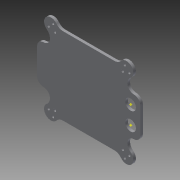
# Autodesk Inventor part: LowerPlatter
Saved by Autodesk Inventor 2015 (Build 190159000, 159)
## iProperties
Created: 2015-06-01
Part Number: LowerPlatter
Material: ABS Plastic
Document SubType Name: Modeling
Designer: Vu
Density: 1.06 g/cm^3
Appearance: Smooth - White
Mass: 73.1056 g
Surface Area: 379.193 cm^2
Volume: 68.9676 cm^3
Author: Vu
Autodesk Inventor part; units mm, degrees
ref_plane "YZ Plane" through (0, 0, 0) normal (1, 0, 0) x (0, 1, 0)
ref_plane "XZ Plane" through (0, 0, 0) normal (0, 1, 0) x (-1, 0, 0)
ref_plane "XY Plane" through (0, 0, 0) normal (0, 0, 1) x (1, 0, 0)
sketch "Sketch1" plane through (0, 0, 0) normal (0, 1, 0) x (-1, 0, 0)
  line L0 (-0.0023, 59.9989) -> (-40.0023, 59.9989)
  line L1 (-0.0023, 59.9989) -> (39.9977, 59.9989) construction
  line L2 (-60.0163, -0.0152) -> (-60.0163, 39.9848)
  line L3 (-60.0163, -0.0152) -> (-20.0163, -0.0152) construction
  line L4 (-60.0163, -0.0152) -> (-0.0023, -0.0152)
  line L5 (-0.0023, -0.0152) -> (-0.0023, 59.9989)
  arc A0 (-49.9687, 64.958) -> (-40.0023, 59.9989) centre (-40.0023, 72.4933) ccw
  arc A1 (-60.0163, 39.9848) -> (-64.9755, 49.9513) centre (-72.5108, 39.9848) ccw
  arc A2 (-49.9687, 64.958) -> (-64.9755, 49.9513) centre (-58.5144, 58.4969) ccw
  line L6 (-40.0023, 59.9989) -> (-40.0023, 59.4989)
  line L7 (-60.0163, 39.9848) -> (-59.5163, 39.9848)
  arc A3 (-59.5163, 39.9848) -> (-40.0023, 59.4989) centre (-59.5163, 59.4989) ccw
  line L8 (-60.0163, -0.0152) -> (-80.0163, -0.0152)
  line L9 (-80.0163, -0.0152) -> (-80.0163, 19.9848)
  arc A4 (-70, 30.0011) -> (-60.0163, 39.9848) centre (-70, 39.9848) ccw
  arc A5 (-70, 30.0011) -> (-80.0163, 19.9848) centre (-70, 19.9848) ccw
  line L10 (-60.0163, -40.0152) -> (-59.5163, -40.0152)
  arc A6 (-64.9755, -49.9816) -> (-60.0163, -40.0152) centre (-72.5108, -40.0152) ccw
  line L11 (-60.0163, -0.0152) -> (-60.0163, -40.0152)
  arc A7 (-64.9755, -49.9816) -> (-49.9687, -64.9884) centre (-58.5144, -58.5273) ccw
  arc A8 (-40.0023, -60.0292) -> (-49.9687, -64.9884) centre (-40.0023, -72.5237) ccw
  arc A9 (-40.0023, -59.5292) -> (-59.5163, -40.0152) centre (-59.5163, -59.5292) ccw
  line L12 (-40.0023, -60.0292) -> (-40.0023, -59.5292)
  line L13 (-0.0023, -60.0292) -> (-40.0023, -60.0292)
  line L14 (-0.0023, -0.0152) -> (-0.0023, -60.0292)
  arc A10 (-60.0163, -40.0152) -> (-70, -30.0315) centre (-70, -40.0152) ccw
  line L15 (-80.0163, -0.0152) -> (-80.0163, -20.0152)
  arc A11 (-80.0163, -20.0152) -> (-70, -30.0315) centre (-70, -20.0152) ccw
  arc A12 (80.0118, 19.9848) -> (69.9955, 30.0011) centre (69.9955, 19.9848) ccw
  line L16 (60.0118, -0.0152) -> (80.0118, -0.0152)
  line L17 (80.0118, -0.0152) -> (80.0118, 19.9848)
  line L18 (-0.0023, 59.9989) -> (-40.0023, 59.9989) construction
  line L19 (-0.0023, 59.9989) -> (39.9977, 59.9989)
  line L20 (60.0118, -0.0152) -> (60.0118, 39.9848)
  arc A13 (60.0118, 39.9848) -> (69.9955, 30.0011) centre (69.9955, 39.9848) ccw
  line L21 (60.0118, 39.9848) -> (59.5118, 39.9848)
  arc A14 (64.9709, 49.9513) -> (60.0118, 39.9848) centre (72.5063, 39.9848) ccw
  line L22 (60.0118, -0.0152) -> (20.0118, -0.0152) construction
  arc A15 (64.9709, 49.9513) -> (49.9642, 64.958) centre (58.5098, 58.4969) ccw
  arc A16 (39.9977, 59.4989) -> (59.5118, 39.9848) centre (59.5118, 59.4989) ccw
  line L23 (39.9977, 59.9989) -> (39.9977, 59.4989)
  arc A17 (39.9977, 59.9989) -> (49.9642, 64.958) centre (39.9977, 72.4933) ccw
  line L24 (60.0118, -0.0152) -> (-0.0023, -0.0152)
  line L25 (80.0118, -0.0152) -> (80.0118, -20.0152)
  arc A18 (69.9955, -30.0315) -> (80.0118, -20.0152) centre (69.9955, -20.0152) ccw
  arc A19 (69.9955, -30.0315) -> (60.0118, -40.0152) centre (69.9955, -40.0152) ccw
  line L26 (60.0118, -40.0152) -> (59.5118, -40.0152)
  line L27 (60.0118, -0.0152) -> (60.0118, -40.0152)
  arc A20 (60.0118, -40.0152) -> (64.9709, -49.9816) centre (72.5063, -40.0152) ccw
  arc A21 (59.5118, -40.0152) -> (39.9977, -59.5292) centre (59.5118, -59.5292) ccw
  arc A22 (49.9642, -64.9884) -> (64.9709, -49.9816) centre (58.5098, -58.5273) ccw
  line L28 (39.9977, -60.0292) -> (39.9977, -59.5292)
  arc A23 (49.9642, -64.9884) -> (39.9977, -60.0292) centre (39.9977, -72.5237) ccw
  line L29 (-0.0023, -60.0292) -> (39.9977, -60.0292)
  point P0 (0, 0)
  point P1 (-55.5, 62.5)
  point P2 (-62.5, 55.5)
  point P3 (-52.5, 52.5)
  point P4 (-52.5, -52.5303)
  point P5 (-62.5, -55.5303)
  point P6 (-55.5, -62.5303)
  point P7 (55.4955, -62.5303)
  point P8 (62.4955, -55.5303)
  point P9 (52.4955, -52.5303)
  point P10 (52.4955, 52.5)
  point P11 (62.4955, 55.5)
  point P12 (55.4955, 62.5)
  point P13 (-65, 13.9848)
  point P14 (-65, -14.0152)
  dimension "d0" = 40
  dimension "d1" = 180
  dimension "d2" = 40
  dimension "d3" = 90
  dimension "d4" = 12.4944
  dimension "d5" = 12.4944
  dimension "d6" = 0.5
  dimension "d7" = 0.5
  dimension "d8" = 20
  dimension "d9" = 20
  dimension "d42" = 14
  dimension "d43" = 14
  constraints: 60 end point, 56 symmetric about line, 48 point on circle, 24 centre point, 9 tangent, 6 horizontal, 2 equal length, 2 perpendicular, 2 vertical, 18 other
  measures "d0" distance of L0.start L0.end
  measures "d1" angle of L0 L1
  measures "d2" distance of L3.start L2.end
  measures "d3" angle of L3 L2
  measures "d4" radius of A0
  measures "d5" radius of A1
  measures "d6" distance of L0.end L6.end
  measures "d7" distance of L2.end L7.end
  measures "d8" distance of L3.start L8.end
  measures "d9" distance of L8.end L9.end
  measures "d42" distance from line of L8 point (-65, 13.985)
  measures "d43" distance from line of point (-65, -14.015) L8
extrude "Extrusion1" add sketch "Sketch1" along normal blind 4 contours L5 L4 L2 L7 A3 L6 L0 | L19 L23 A16 L21 L20 L24 L5 | L14 L13 L12 A9 L10 L11 L4 | L24 L27 L26 A21 L28 L29 L14 | L8 L9 A5 A4 L2 | L11 A10 A11 L15 L8 | L20 A13 A12 L17 L16 | L16 L25 A18 A19 L27
extrude "Extrusion2" add sketch "Sketch1" along normal blind 4 contours L6 A3 L7 A1 A2 A0 | A17 A15 A14 L21 A16 L23 | L10 A9 L12 A8 A7 A6 | L28 A21 L26 A20 A22 A23
hole "Hole1" at (65, 0, -14.0152) direction (0, 1, 0) diameter 16.5 end through all
hole "Hole2" at (65, 0, 13.9848) direction (0, 1, 0) diameter 16.5 end through all
hole "Hole3" at (-55.4955, 0, 62.5) at (-62.4955, 0, 55.5) at (-52.4955, 0, 52.5) at (-52.4955, 0, -52.5303) at (-62.4955, 0, -55.5303) at (-55.4955, 0, -62.5303) at (55.5, 0, -62.5303) at (62.5, 0, -55.5303) at (52.5, 0, -52.5303) at (52.5, 0, 52.5) at (62.5, 0, 55.5) at (55.5, 0, 62.5) at (65, 0, 13.9848) at (65, 0, -14.0152) direction (0, 1, 0) diameter 4 end through all
body "Solid1"
